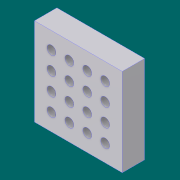
# Autodesk Inventor part: L1F2-U
Saved by Autodesk Inventor 2016 (Build 200138000, 138)
## iProperties
Created: 2016-02-09
Part Number: L1F2-U
Material: Glass
Document SubType Name: Modeling
Designer: Sawaiz
Density: 2.18 g/cm^3
Appearance: Cool White
Author: Sawaiz
Autodesk Inventor part; units mm, degrees
ref_plane "YZ Plane" through (0, 0, 0) normal (1, 0, 0) x (0, 1, 0)
ref_plane "XZ Plane" through (0, 0, 0) normal (0, 1, 0) x (-1, 0, 0)
ref_plane "XY Plane" through (0, 0, 0) normal (0, 0, 1) x (1, 0, 0)
sketch "Sketch1" plane through (0, 0, 0) normal (1, 0, 0) x (0, 1, 0)
  line L0 (-0.49, 0.49) -> (0.49, 0.49)
  line L1 (0.49, 0.49) -> (0.49, -0.49)
  line L2 (0.49, -0.49) -> (-0.49, -0.49)
  line L3 (-0.49, -0.49) -> (-0.49, 0.49)
  line L4 (-0.49, 0.49) -> (0.49, -0.49) construction
  line L5 (0.49, 0.49) -> (-0.49, -0.49) construction
  point P0 (0, 0)
  dimension "d0" = 0.98
  dimension "d1" = 0.98
  constraints: 12 end point, 2 midpoint, 2 parallel, 1 horizontal, 1 perpendicular
  measures "d0" distance of L1.end L2.end
  measures "d1" distance of L0.end L1.end
extrude "Extrusion1" add sketch "Sketch1" along normal blind 0.25
sketch "Sketch2" plane through (0.25, 0, 0) normal (1, 0, 0) x (0, 0, -1)
  circle A0 centre (-0.3, -0.3) radius 0.05
  point P0 (0, 0)
  dimension "d4" = 0.1
  dimension "d5" = 0.3
  dimension "d6" = 0.3
  constraints: 1 centre point
  measures "d4" diameter of A0
  measures "d5" horizontal distance of A0.centre point (0, 0)
  measures "d6" horizontal distance of A0.centre point (0, 0)
extrude "Extrusion2" cut sketch "Sketch2" against normal blind 0.05
fillet "Fillet1" radius 0.05 1 edges at (0.2, -0.3, 0.35)
pattern_linear "Rectangular Pattern1" count 4 spacing 0.2 along (0, 1, 0) count 4 spacing 0.2 along (0, 0, -1) of "Extrusion2", "Fillet1"
sketch "Sketch3" plane through (0, 0, 0) normal (-1, 0, 0) x (0, 0, 1)
  line L0 (0.49, -0.49) -> (0.49, 0.49) projected
  line L1 (0.49, 0.49) -> (-0.49, 0.49) projected
  line L2 (-0.49, 0.49) -> (-0.49, -0.49) projected
  line L3 (-0.49, -0.49) -> (0.49, -0.49) projected
  line L4 (0.47, 0.47) -> (-0.47, 0.47)
  line L5 (-0.47, 0.47) -> (-0.47, 0.1)
  line L6 (-0.47, 0.1) -> (0.47, 0.1)
  line L7 (0.47, 0.1) -> (0.47, 0.47)
  line L8 (-0.47, -0.1) -> (0.47, -0.1)
  line L9 (0.47, -0.1) -> (0.47, -0.47)
  line L10 (0.47, -0.47) -> (-0.47, -0.47)
  line L11 (-0.47, -0.47) -> (-0.47, -0.1)
  line L12 (0, 0.1) -> (0, 0)
  dimension "d16" = 0.2
  dimension "d17" = 0.37
  dimension "d18" = 0.37
  dimension "d19" = 0.94
  dimension "d20" = 0.02
  dimension "d21" = 0.1
  constraints: 18 end point, 4 parallel, 2 horizontal, 2 perpendicular, 2 point on line, 1 midpoint
  measures "d16" distance between parallel lines of L8 L6
  measures "d17" distance of L4.end L5.end
  measures "d18" distance of L10.end L8.start
  measures "d19" distance of L9.end L10.end
  measures "d20" distance between parallel lines of L0 L9
  measures "d21" distance of L12.start L12.end
extrude "Extrusion3" add sketch "Sketch3" along normal blind 0.01 separate body contours L7 L6 L5 L4 | L8 L9 L10 L11
equation "\"d21\" = 0.5 * d16"
body "Solid1"
body "Solid2"
